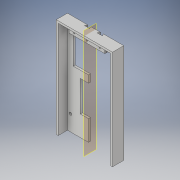
# Autodesk Inventor part: foot_cover_2_bottom
Saved by Autodesk Inventor 2018 (Build 220112000, 112)
## iProperties
Created: 2018-12-11
Part Number: foot_cover_2_bottom
Material: Generic
Document SubType Name: Modeling
Designer: jaspe
Density: 1 g/cm^3
Appearance: Default
Author: jaspe
Autodesk Inventor part; units mm, degrees
ref_plane "YZ Plane" through (0, 0, 0) normal (1, 0, 0) x (0, 1, 0)
ref_plane "XZ Plane" through (0, 0, 0) normal (0, 1, 0) x (-1, 0, 0)
ref_plane "XY Plane" through (0, 0, 0) normal (0, 0, 1) x (1, 0, 0)
sketch "Sketch1" plane through (0, 0, 0) normal (0, 1, 0) x (-1, 0, 0)
  line L0 (-55, 100) -> (55, 100)
  line L1 (55, 100) -> (55, -100)
  line L2 (55, -100) -> (-55, -100)
  line L3 (-55, -100) -> (-55, 100)
  line L4 (-55, 100) -> (55, -100) construction
  line L5 (55, 100) -> (-55, -100) construction
  point P0 (0, 0)
  dimension "d0" = 110
  dimension "d1" = 200
  constraints: 12 end point, 2 midpoint, 2 parallel, 1 horizontal, 1 perpendicular
  measures "d0" distance of L1.end L2.end
  measures "d1" distance of L0.end L1.end
extrude "Extrusion1" add sketch "Sketch1" along normal blind 22
sketch "Sketch2" plane through (0, 22, 0) normal (0, 1, 0) x (1, 0, 0)
  line L0 (55, -100) -> (55, 100) construction
  line L1 (55, 100) -> (40, 100) construction
  line L2 (55, 100) -> (-55, 100) construction
  line L3 (55, 100) -> (70, 100) construction
  line L4 (40, 100) -> (-10, 100)
  line L5 (-10, 100) -> (-10, -20)
  line L6 (-10, -20) -> (40, -20)
  line L7 (40, -20) -> (40, 100)
  point P0 (0, 0)
  dimension "d4" = 15
  dimension "d5" = 180
  dimension "d6" = 50
  dimension "d7" = 120
  constraints: 12 end point, 2 collinear, 2 horizontal, 2 parallel, 1 perpendicular
  measures "d4" distance of L0.end L1.end
  measures "d5" angle of L1 L3
  measures "d6" distance of L6.end L5.end
  measures "d7" distance of L5.end L4.end
sketch "Sketch3" plane through (0, 0, 0) normal (0, -1, 0) x (1, 0, 0)
  line L0 (-51, 96) -> (51, 96)
  line L1 (51, 96) -> (51, -96)
  line L2 (51, -96) -> (-51, -96)
  line L3 (-51, -96) -> (-51, 96)
  line L4 (-51, 96) -> (51, -96) construction
  line L5 (51, 96) -> (-51, -96) construction
  point P0 (0, 0)
  dimension "d8" = 102
  dimension "d9" = 192
  constraints: 12 end point, 2 midpoint, 2 parallel, 1 horizontal, 1 perpendicular
  measures "d8" distance of L1.end L2.end
  measures "d9" distance of L0.end L1.end
extrude "Extrusion2" cut sketch "Sketch3" against normal blind 18
extrude "Extrusion3" cut sketch "Sketch2" against normal up to surface (22 mm away)
sketch "Sketch4" plane through (0, 22, 0) normal (0, 1, 0) x (1, 0, 0)
  line L0 (40, -20) -> (-10, -20) projected
  line L1 (40, -20) -> (-40, -20)
  line L2 (-40, -20) -> (-40, -85)
  line L3 (-40, -85) -> (40, -85)
  line L4 (40, -85) -> (40, -20)
  point P0 (0, 0)
  dimension "d14" = 80
  dimension "d15" = 65
  constraints: 8 end point, 2 parallel, 1 horizontal, 1 perpendicular
  measures "d14" distance of L3.end L2.end
  measures "d15" distance of L2.end L1.end
extrude "Extrusion4" cut sketch "Sketch4" against normal blind 13
sketch "Sketch6" plane through (0, 22, 0) normal (0, 1, 0) x (1, 0, 0)
  line L0 (40, 100) -> (40, -85) projected
  line L1 (40, -85) -> (-40, -85) projected
  line L2 (-40, -85) -> (-40, -20) projected
  line L3 (-40, -20) -> (-10, -20) projected
  line L4 (-10, -20) -> (-10, 100) projected
  line L5 (-10, 100) -> (-55, 100) projected
  line L6 (-55, 100) -> (-55, -100) projected
  line L7 (-55, -100) -> (55, -100) projected
  line L8 (55, -100) -> (55, 100) projected
  line L9 (55, 100) -> (40, 100) projected
  line L10 (-55, 100) -> (-55, 63) construction
  line L11 (-55, 100) -> (-18, 100) construction
  line L12 (-55, 63) -> (-45, 63) construction
  circle A0 centre (-45, 63) radius 2.5
  line L13 (55, 100) -> (55, -100) construction
  line L14 (55, 100) -> (55, 63) construction
  line L15 (55, 100) -> (92, 100) construction
  line L16 (55, 63) -> (45, 63) construction
  circle A1 centre (45, 63) radius 2.5
  point P0 (0, 0)
  dimension "d24" = 37
  dimension "d25" = 90
  dimension "d26" = 10
  dimension "d27" = 90
  dimension "d28" = 5
  dimension "d29" = 37
  dimension "d30" = 90
  dimension "d31" = 10
  dimension "d32" = 90
  dimension "d33" = 5
  constraints: 12 end point, 4 perpendicular, 2 centre point, 2 coincident, 2 horizontal, 1 collinear, 1 vertical
  measures "d24" distance of L5.end L10.end
  measures "d25" angle of L10 L11
  measures "d26" distance of L10.end L12.end
  measures "d27" angle of L12 L10
  measures "d28" diameter of A0
  measures "d29" distance of L8.end L14.end
  measures "d30" angle of L14 L15
  measures "d31" distance of L14.end L16.end
  measures "d32" angle of L14 L16
  measures "d33" diameter of A1
extrude "Extrusion6" cut sketch "Sketch6" against normal blind 10 contours A0 | A1
sketch "Sketch8" plane through (0, 18, 0) normal (0, -1, 0) x (1, 0, 0)
  line L0 (51, 96) -> (51, -96) construction
  line L1 (51, 96) -> (35, 96) construction
  line L2 (-51, 96) -> (51, 96) construction
  line L3 (51, 96) -> (67, 96) construction
  line L4 (35, 96) -> (-35, 96)
  line L5 (-35, 96) -> (-35, 85)
  line L6 (-35, 85) -> (35, 85)
  line L7 (35, 85) -> (35, 96)
  point P0 (0, 0)
  dimension "d57" = 16
  dimension "d58" = 180
  dimension "d59" = 70
  dimension "d60" = 11
  constraints: 12 end point, 2 collinear, 2 horizontal, 2 parallel, 1 perpendicular
  measures "d57" distance of L0.start L1.end
  measures "d58" angle of L1 L3
  measures "d59" distance of L6.end L5.end
  measures "d60" distance of L5.end L4.end
extrude "Extrusion8" add sketch "Sketch8" along normal blind 13
sketch "Sketch7" plane through (-55, 0, 100) normal (0, 0, 1) x (1, 0, 0)
  line L0 (45, 22) -> (0, 22) construction
  line L1 (0, 22) -> (39.8, 22) construction
  line L2 (39.8, 22) -> (37.3, 17.6699)
  line L3 (39.8, 22) -> (44.8, 22) construction
  line L4 (37.3, 17.6699) -> (47.7, 17.6699)
  line L5 (45, 18) -> (4, 18) projected
  line L6 (47.7, 17.6699) -> (45.2, 22)
  line L7 (15, 22) -> (45, 22) projected
  line L8 (45.2, 22) -> (39.8, 22)
  line L9 (0, 22) -> (110, 22) projected
  line L10 (110, 22) -> (70.2, 22)
  line L11 (110, 22) -> (149.8, 22) construction
  line L12 (70.2, 22) -> (72.7, 17.6699)
  line L13 (72.7, 17.6699) -> (62.3, 17.6699)
  line L14 (15, 18) -> (95, 18) projected
  line L15 (62.3, 17.6699) -> (64.8, 22)
  line L16 (64.8, 22) -> (70.2, 22)
  point P0 (55, 0)
  dimension "d36" = 39.8
  dimension "d39" = 5
  dimension "d40" = 120
  dimension "d41" = 10.4
  dimension "d42" = 60
  dimension "d43" = 5
  dimension "d44" = 60
  dimension "d45" = 5.4
  dimension "d46" = 120
  dimension "d47" = 39.8
  dimension "d48" = 180
  dimension "d49" = 5
  dimension "d50" = 60
  dimension "d51" = 10.4
  dimension "d52" = 60
  dimension "d53" = 5
  dimension "d54" = 60
  constraints: 24 end point, 2 equal length, 2 horizontal, 2 parallel, 1 collinear, 1 point on line
  measures "d36" distance of L0.end L1.end
  measures "d39" distance of L1.end L2.end
  measures "d40" angle of L2 L3
  measures "d41" distance of L2.end L4.end
  measures "d42" angle of L4 L2
  measures "d43" distance of L4.end L6.end
  measures "d44" angle of L6 L4
  measures "d45" distance of L6.end L1.end
  measures "d46" angle of L8 L6
  measures "d47" distance of L9.end L10.end
  measures "d48" angle of L10 L11
  measures "d49" distance of L10.end L12.end
  measures "d50" angle of L12 L10
  measures "d51" distance of L12.end L13.end
  measures "d52" angle of L12 L13
  measures "d53" distance of L13.end L15.end
  measures "d54" angle of L13 L15
extrude "Extrusion7" cut sketch "Sketch7" against normal blind 6 contours L7 L8 L6 L14 L5 L2 | L5 L14 L6 L4 L2 | L9 L12 L14 L15 | L14 L12 L13 L15
sketch "Sketch9" plane through (0, 0, 0) normal (0, -1, 0) x (1, 0, 0)
  line L0 (-10, -100) -> (-10, -96) projected
  line L1 (-10, -96) -> (-51, -96) projected
  line L2 (-51, -96) -> (-51, 96) projected
  line L3 (-51, 96) -> (51, 96) projected
  line L4 (51, 96) -> (51, -96) projected
  line L5 (51, -96) -> (40, -96) projected
  line L6 (40, -96) -> (40, -100) projected
  line L7 (40, -100) -> (55, -100) projected
  line L8 (55, -100) -> (55, 100) projected
  line L9 (55, 100) -> (-55, 100) projected
  line L10 (-55, 100) -> (-55, -100) projected
  line L11 (-55, -100) -> (-10, -100) projected
  line L12 (55, 100) -> (-55, 100) projected
  line L13 (0, 100) -> (0, 90)
  line L14 (0, 100) -> (10, 100) construction
  line L15 (0, 90) -> (-25, 90)
  line L16 (0, 90) -> (25, 90)
  circle A0 centre (25, 90) radius 1.5
  circle A1 centre (0, 90) radius 1.5
  circle A2 centre (-25, 90) radius 1.5
  point P0 (0, 0)
  dimension "d63" = 10
  dimension "d64" = 90
  dimension "d65" = 25
  dimension "d66" = 180
  dimension "d67" = 3
  dimension "d68" = 3
  dimension "d69" = 3
  constraints: 8 end point, 3 centre point, 3 coincident, 3 horizontal, 2 equal length, 1 midpoint, 1 vertical
  measures "d63" distance of L13.start L13.end
  measures "d64" angle of L13 L14
  measures "d65" distance of L13.end L15.end
  measures "d66" angle of L15 L16
  measures "d67" diameter of A0
  measures "d68" diameter of A1
  measures "d69" diameter of A2
extrude "Extrusion9" cut sketch "Sketch9" against normal blind 10 contours A0 | A2 | A1 L16 L13 | L13 L15 A1 | L16 A1 L15
sketch "Sketch10" plane through (-55, 0, -100) normal (0, 0, -1) x (-1, 0, 0)
  line L0 (-45, 22) -> (-45, 0) projected
  line L1 (0, 0) -> (-45, 0) projected
  line L2 (0, 0) -> (0, 22) projected
  line L3 (-45, 22) -> (0, 22) projected
  line L4 (-95, 0) -> (-95, 22) projected
  line L5 (-110, 22) -> (-95, 22) projected
  line L6 (-110, 0) -> (-110, 22) projected
  line L7 (-95, 0) -> (-110, 0) projected
  line L8 (0, 0) -> (-110, 0)
  line L9 (-110, 0) -> (-110, 22)
  line L10 (-110, 22) -> (0, 22)
  line L11 (0, 22) -> (0, 0)
  point P0 (-55, 0)
  constraints: 8 end point, 2 parallel, 1 horizontal, 1 perpendicular
extrude "Extrusion11" cut sketch "Sketch10" against normal blind 6 contours L3 L2 L1 L0 | L4 L7 L6 L5
sketch "Sketch11" plane through (0, 22, 0) normal (0, 1, 0) x (1, 0, 0)
  line L0 (-10, -20) -> (-40, -20) construction
  line L1 (-10, -20) -> (-10, -6) construction
  line L2 (-10, 94) -> (-10, -20) construction
  line L3 (-10, -6) -> (-26, -6)
  line L4 (-26, -6) -> (-26, 54)
  line L5 (-26, 54) -> (-10, 54)
  line L6 (-10, 54) -> (-10, -6)
  line L7 (-10, -6) -> (40, -6) construction
  line L8 (40, -85) -> (40, 94) construction
  line L9 (40, -6) -> (50, -6)
  line L10 (50, -6) -> (50, 54)
  line L11 (50, 54) -> (40, 54)
  line L12 (40, 54) -> (40, -6)
  point P0 (0, 0)
  dimension "d77" = 14
  dimension "d78" = 16
  dimension "d79" = 60
  dimension "d80" = 10
  dimension "d81" = 60
  constraints: 20 end point, 4 parallel, 3 horizontal, 2 perpendicular, 2 point on line
  measures "d77" distance of L0.start L1.end
  measures "d78" distance of L4.end L5.end
  measures "d79" distance of L3.end L4.end
  measures "d80" distance of L11.end L10.end
  measures "d81" distance of L10.end L9.end
extrude "Extrusion12" cut sketch "Sketch11" against normal up to surface (4 mm away)
ref_plane "Work Plane1" through (0, 0, 100) normal (1, 0, 0) x (0, 0, -1)
body "Solid1"
